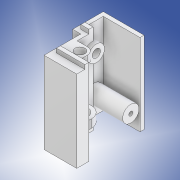
# Autodesk Inventor part: BA003
Saved by Autodesk Inventor 2017 SP1 (Build 210196100, 196)
## iProperties
Created: 2017-06-15
Part Number: BA003
Material: ABS Plastic
Document SubType Name: Modeling
Designer: zallen
Density: 1.06 g/cm^3
Appearance: CR White
Author: zallen
Autodesk Inventor part; units mm, degrees
ref_plane "YZ Plane" through (0, 0, 0) normal (1, 0, 0) x (0, 1, 0)
ref_plane "XZ Plane" through (0, 0, 0) normal (0, 1, 0) x (-1, 0, 0)
ref_plane "XY Plane" through (0, 0, 0) normal (0, 0, 1) x (1, 0, 0)
sketch "Sketch1" plane through (0, 0, 0) normal (0, 0, 1) x (1, 0, 0)
  line L0 (0, 0) -> (40, 0)
  line L1 (40, 0) -> (40, 100)
  line L2 (40, 100) -> (0, 100)
  line L3 (0, 100) -> (0, 0)
  dimension "d0" = 40
  dimension "d1" = 100
  constraints: 8 end point, 2 parallel, 1 horizontal, 1 perpendicular
  measures "d0" distance of L2.end L1.end
  measures "d1" distance of L1.end L0.end
extrude "Extrusion1" add sketch "Sketch1" along normal blind 45
sketch "Sketch2" plane through (0, 0, 0) normal (0, 0, -1) x (-1, 0, 0)
  line L0 (-40, 0) -> (-40, 100) projected
  line L1 (-40, 100) -> (10, 100)
  line L2 (10, 100) -> (10, 0)
  line L3 (10, 0) -> (-40, 0)
  line L4 (-40, 0) -> (-40, 100)
  point P0 (0, 0)
  dimension "d4" = 10
  constraints: 8 end point, 2 parallel, 1 horizontal, 1 horizontal alignment, 1 perpendicular
  measures "d4" distance from line of point (0, 0) L2
extrude "Extrusion2" add sketch "Sketch2" along normal blind 37.5
sketch "Sketch3" plane through (40, 0, 45) normal (1, 0, 0) x (0, 0, -1)
  line L0 (82.5, 100) -> (0, 100) projected
  line L1 (0, 0) -> (0, 100) projected
  line L2 (82.5, 0) -> (0, 0) projected
  line L3 (82.5, 100) -> (82.5, 0) projected
  line L4 (5, 5) -> (5, 95)
  line L5 (5, 95) -> (77.5, 95)
  line L6 (77.5, 95) -> (77.5, 5)
  line L7 (77.5, 5) -> (5, 5)
  point P0 (45, 0)
  dimension "d7" = 5
  constraints: 8 end point, 3 other
  measures "d7" distance between parallel lines of L2 L7
extrude "Extrusion3" cut sketch "Sketch3" against normal blind 35 contours L4 L5 L6 L7
sketch "Sketch4" plane through (5, 0, 45) normal (1, 0, 0) x (0, 0, -1)
  line L0 (45, 100) -> (45, 0) projected
  line L1 (45, 100) -> (82.5, 100) projected
  line L2 (82.5, 0) -> (82.5, 100) projected
  line L3 (45, 0) -> (82.5, 0) projected
  line L4 (50, 5) -> (50, 95)
  line L5 (50, 95) -> (77.5, 95)
  line L6 (77.5, 95) -> (77.5, 5)
  line L7 (77.5, 5) -> (50, 5)
  point P0 (45, 0)
  dimension "d10" = 5
  constraints: 8 end point, 3 other
  measures "d10" distance between parallel lines of L0 L4
extrude "Extrusion4" cut sketch "Sketch4" against normal blind 10 contours L4 L5 L6 L7
sketch "Sketch5" plane through (0, 0, 45) normal (0, -1, 0) x (1, 0, 0)
  line L0 (0, 0) -> (40, 0) projected
  line L1 (0, -45) -> (0, 0) projected
  line L2 (-10, -45) -> (0, -45) projected
  line L3 (-10, -45) -> (-10, -82.5) projected
  line L4 (40, -82.5) -> (-10, -82.5) projected
  line L5 (40, -77.5) -> (-5, -77.5)
  line L6 (-5, -77.5) -> (-5, -50)
  line L7 (-5, -50) -> (5, -50)
  line L8 (5, -50) -> (5, -5)
  line L9 (5, -5) -> (40, -5)
  line L10 (40, -77.5) -> (40, -5)
  line L11 (40, -82.5) -> (40, 0) projected
  dimension "d13" = 5
  constraints: 12 end point, 1 collinear, 4 other
  measures "d13" distance between parallel lines of L4 L5
extrude "Extrusion5" cut sketch "Sketch5" against normal through all contours L10 L5 L6 L7 L8 L9
sketch "Sketch6" plane through (0, 100, 45) normal (0, 1, 0) x (1, 0, 0)
  line L0 (0, 45) -> (0, 0) projected
  line L1 (0, 0) -> (40, 0)
  line L2 (40, 0) -> (40, 10)
  line L3 (40, 10) -> (0, 10)
  line L4 (0, 10) -> (0, 0)
  dimension "d16" = 40
  dimension "d17" = 10
  constraints: 8 end point, 2 parallel, 1 horizontal, 1 perpendicular
  measures "d16" distance of L3.end L2.end
  measures "d17" distance of L2.end L1.end
extrude "Extrusion6" add sketch "Sketch6" against normal blind 100
sketch "Sketch8" plane through (40, 100, 35) normal (0, 0, -1) x (-1, 0, 0)
  line L0 (35, 0) -> (35, -100) projected
  line L1 (0, 0) -> (35, 0) projected
  line L2 (0, 0) -> (0, -100) projected
  line L3 (35, -100) -> (0, -100) projected
  line L4 (35, -105) -> (0, -105)
  line L5 (0, -105) -> (0, 5)
  line L6 (0, 5) -> (35, 5)
  line L7 (35, 5) -> (35, -105)
  point P0 (40, -100)
  dimension "d20" = 5
  dimension "d21" = 5
  constraints: 8 end point, 2 parallel, 1 horizontal, 1 perpendicular, 1 point on line
  measures "d20" distance between parallel lines of L4 L3
  measures "d21" distance between parallel lines of L1 L6
extrude "Extrusion7" add sketch "Sketch8" along normal blind 5
sketch "Sketch10" plane through (5, 0, -5) normal (0, 0, -1) x (-1, 0, 0)
  line L0 (0, 0) -> (0, 100) projected
  line L1 (10, 0) -> (0, 0) projected
  line L2 (10, 0) -> (10, 100) projected
  line L3 (0, 100) -> (10, 100) projected
  line L4 (-35, -5) -> (0, -5) projected
  line L5 (10, 0) -> (0, 0)
  line L6 (0, 0) -> (0, -5)
  line L7 (0, -5) -> (10, -5)
  line L8 (10, -5) -> (10, 0)
  line L9 (0, 105) -> (0, 100) projected
  line L10 (10, 100) -> (0, 100)
  line L11 (0, 100) -> (0, 105)
  line L12 (0, 105) -> (10, 105)
  line L13 (10, 105) -> (10, 100)
  point P0 (5, 0)
  constraints: 16 end point, 4 parallel, 2 horizontal, 2 perpendicular
extrude "Extrusion8" add sketch "Sketch10" along normal blind 5
sketch "Sketch25" plane through (5, 0, 45) normal (1, 0, 0) x (0, 0, -1)
  circle A0 centre (32.5, 25) radius 10
  circle A1 centre (32.5, 25) radius 2.5
  line L0 (50, 0) -> (15, 0) projected
  line L1 (15, 105) -> (15, -5) projected
  circle A2 centre (66.25, 25) radius 2.5
  circle A3 centre (66.25, 25) radius 10
  line L2 (77.5, 0) -> (55, 0) projected
  point P0 (32.5, 0)
  point P1 (15, 55)
  point P2 (15, 25)
  point P3 (66.25, 0)
  dimension "d89" = 20
  dimension "d90" = 5
  dimension "d93" = 5
  dimension "d94" = 20
  constraints: 4 centre point, 2 coincident, 2 horizontal alignment, 2 midpoint, 2 vertical alignment, 1 point on line
  measures "d89" diameter of A0
  measures "d90" diameter of A1
  measures "d93" diameter of A2
  measures "d94" diameter of A3
extrude "Extrusion22" add sketch "Sketch25" along normal blind 35 contours A3
sketch "Sketch26" plane through (-5, 0, 45) normal (1, 0, 0) x (0, 0, -1)
  circle A0 centre (66.25, 25) radius 10 projected
  circle A1 centre (66.25, 25) radius 2.5 projected
  point P0 (45, 0)
extrude "Extrusion23" add sketch "Sketch26" along normal blind 10
sketch "Sketch27" plane through (5, 0, 45) normal (1, 0, 0) x (0, 0, -1)
  circle A0 centre (54, 80) radius 10
  circle A1 centre (54, 80) radius 5
  line L0 (15, 105) -> (15, -5) projected
  line L1 (15, 100) -> (50, 100) projected
  point P0 (45, 0)
  dimension "d98" = 20
  dimension "d99" = 10
  dimension "d100" = 39
  dimension "d101" = 20
  constraints: 2 centre point, 1 coincident
  measures "d98" diameter of A0
  measures "d99" diameter of A1
  measures "d100" distance from line of L0 A0.centre
  measures "d101" distance from line of L1 A0.centre
extrude "Extrusion24" add sketch "Sketch27" along normal blind 5
sketch "Sketch28" plane through (-5, 0, 45) normal (1, 0, 0) x (0, 0, -1)
  circle A0 centre (54, 80) radius 5 projected
  circle A1 centre (54, 80) radius 10 projected
  line L0 (54, 70) -> (54, 90)
  point P0 (45, 0)
  constraints: 2 end point, 2 point on circle, 1 vertical
extrude "Extrusion25" add sketch "Sketch28" along normal blind 10 contours A0 L0 | A0 L0 A1 picked at (56.5956, 79.4001) picked at (62.208, 81.1126)
sketch "Sketch29" plane through (5, 80, -9) normal (1, 0, 0) x (0, 0, -1)
  circle A0 centre (0, 0) radius 5 projected
  point P0 (-9, -80)
extrude "Extrusion26" cut sketch "Sketch29" against normal blind 10
sketch "Sketch30" plane through (40, 0, 45) normal (1, 0, 0) x (0, 0, -1)
  line L0 (10, 0) -> (0, 0) projected
  line L1 (15, -5) -> (15, 0) projected
  line L2 (10, 0) -> (15, 0)
  line L3 (15, 0) -> (15, -5)
  line L4 (15, -5) -> (10, -5)
  line L5 (10, -5) -> (10, 0)
  point P0 (45, 0)
  constraints: 8 end point, 2 parallel, 1 horizontal, 1 perpendicular
extrude "Extrusion27" cut sketch "Sketch30" against normal through all
sketch "Sketch31" plane through (40, 100, 30) normal (0, 0, -1) x (-1, 0, 0)
  line L0 (40, -100) -> (0, -100) projected
  line L1 (0, -100) -> (0, 0) projected
  line L2 (0, 0) -> (40, 0) projected
  line L3 (40, 0) -> (40, -100) projected
  line L4 (10, -95) -> (25, -95)
  line L5 (25, -95) -> (25, -85)
  line L6 (25, -85) -> (10, -85)
  line L7 (10, -85) -> (10, -95)
  line L8 (35, 0) -> (35, -100) projected
  dimension "d110" = 15
  dimension "d111" = 10
  dimension "d112" = 10
  dimension "d113" = 5
  constraints: 8 end point, 2 parallel, 1 horizontal, 1 perpendicular
  measures "d110" distance of L6.end L5.end
  measures "d111" distance of L5.end L4.end
  measures "d112" distance between parallel lines of L1 L7
  measures "d113" distance between parallel lines of L0 L4
extrude "Extrusion28" cut sketch "Sketch31" against normal blind 5 contours L7 L6 L5 L4
fillet "Fillet1" radius 2 4 edges at (15, 10, 30) (30, 10, 30) (15, 10, 35) (30, 10, 35)
sketch "Sketch32" plane through (0, 0, 45) normal (0, -1, 0) x (1, 0, 0)
  line L0 (2, -11) -> (33, -11) construction
  line L1 (33, -11) -> (33, -42) construction
  line L2 (33, -42) -> (2, -42) construction
  line L3 (2, -42) -> (2, -11) construction
  line L4 (40, -82.5) -> (-10, -82.5) construction
  line L5 (40, 0) -> (40, -15) construction
  circle A0 centre (33, -11) radius 2.5
  point P0 (0, -45)
  dimension "d117" = 31
  dimension "d118" = 31
  dimension "d119" = 40.5
  dimension "d120" = 7
  dimension "d121" = 5
  constraints: 8 end point, 2 parallel, 1 centre point, 1 coincident, 1 horizontal, 1 perpendicular
  measures "d117" distance of L1.end L2.end
  measures "d118" distance of L0.end L1.end
  measures "d119" distance between parallel lines of L4 L2
  measures "d120" distance between parallel lines of L5 L1
  measures "d121" diameter of A0
extrude "Extrusion29" cut sketch "Sketch32" against normal blind 5
sketch "Sketch33" plane through (0, 100, 45) normal (0, 1, 0) x (1, 0, 0)
  circle A0 centre (17.5, 26.5) radius 6
  circle A1 centre (17.5, 26.5) radius 9 construction
  line L0 (26.5, 26.5) -> (26.5, 15)
  line L1 (8.5, 15) -> (26.5, 15)
  line L2 (17.5, 35.5) -> (5, 35.5)
  line L3 (5, 15) -> (5, 50) projected
  line L4 (5, 35.5) -> (5, 15)
  line L5 (40, 15) -> (5, 15) projected
  line L6 (5, 15) -> (40, 15) projected
  line L7 (8.5, 15) -> (5, 15)
  arc A2 (26.5, 26.5) -> (17.5, 35.5) centre (17.5, 26.5) ccw
  point P0 (0, 45)
  dimension "d125" = 12
  dimension "d127" = 18
  dimension "d130" = 12.5
  dimension "d131" = 11.5
  constraints: 10 end point, 4 point on circle, 4 tangent, 3 centre point, 3 point on line, 1 coincident, 1 collinear, 1 horizontal, 1 perpendicular, 1 vertical
  measures "d125" diameter of A0
  measures "d127" diameter of A1
  measures "d130" distance from line of L3 A0.centre
  measures "d131" distance from line of L1 A0.centre
extrude "Extrusion32" add sketch "Sketch33" against normal blind 10
sketch "Sketch35" plane through (5, 0, 45) normal (1, 0, 0) x (0, 0, -1)
  circle A0 centre (54, 80) radius 10 projected
  circle A1 centre (54, 80) radius 23
  point P0 (45, 0)
  dimension "d136" = 46
  constraints: 1 centre point, 1 coincident
  measures "d136" diameter of A1
extrude "Extrusion33" cut sketch "Sketch35" along normal through all
ref_plane "Work Plane2" through (0, 25, 45) normal (0, 1, 0) x (1, 0, 0)
sketch "Sketch36" plane through (0, 25, 45) normal (0, 1, 0) x (1, 0, 0)
  line L0 (5, 50) -> (5, 15) projected
  line L1 (5, 15) -> (40, 15) projected
  circle A0 centre (17.5, 26.5) radius 6 construction
  circle A1 centre (17.5, 26.5) radius 9.5
  circle A2 centre (17.5, 26.5) radius 14 construction
  line L2 (31.5, 26.5) -> (31.5, 15)
  line L3 (31.5, 15) -> (5, 15)
  line L4 (5, 40.5) -> (5, 15)
  line L5 (17.5, 40.5) -> (5, 40.5)
  arc A3 (31.5, 26.5) -> (17.5, 40.5) centre (17.5, 26.5) ccw
  point P0 (0, 45)
  dimension "d140" = 19
  dimension "d141" = 28
  constraints: 8 end point, 4 point on circle, 3 centre point, 3 tangent, 2 coincident, 2 collinear, 2 perpendicular, 2 point on line, 1 concentric
  measures "d140" diameter of A1
  measures "d141" diameter of A2
extrude "Extrusion34" add sketch "Sketch36" along normal blind 10
body "Solid1"
